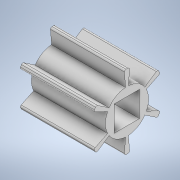
# Autodesk Inventor part: 220411 Small Rod Laddered
Saved by Autodesk Inventor 2022 (Build 260153000, 153)
## iProperties
Created: 2022-01-22
Part Number: 220411 Small Rod Laddered
Material: Generic
Document SubType Name: Modeling
Designer: josephinew
Density: 1 g/cm^3
Appearance: Default
Author: josephinew
Autodesk Inventor part; units mm, degrees
ref_plane "YZ Plane" through (0, 0, 0) normal (1, 0, 0) x (0, 1, 0)
ref_plane "XZ Plane" through (0, 0, 0) normal (0, 1, 0) x (-1, 0, 0)
ref_plane "XY Plane" through (0, 0, 0) normal (0, 0, 1) x (1, 0, 0)
sketch "Sketch1" plane through (0, 0, 0) normal (1, 0, 0) x (0, 1, 0)
  circle A0 centre (0, 0) radius 22.225
  line L0 (13.208, 13.208) -> (-12.954, 13.208)
  line L1 (-12.954, 13.208) -> (-12.954, -12.954)
  line L2 (-12.954, -12.954) -> (13.208, -12.954)
  line L3 (13.208, -12.954) -> (13.208, 13.208)
  dimension "d22" = 44.45
  dimension "d47" = 26.162
  dimension "d48" = 26.162
  constraints: 8 end point, 2 parallel, 1 centre point, 1 horizontal, 1 perpendicular
  measures "d22" diameter of A0
  measures "d47" distance of L2.end L1.end
  measures "d48" distance of L1.end L0.end
extrude "Extrusion1" add sketch "Sketch1" along normal blind 76.2
sketch "Sketch5" plane through (76.2, 0, 0) normal (1, 0, 0) x (0, 0, -1)
  line L0 (0, 0) -> (28.6448, 0) construction
  line L1 (0, 0) -> (30.2362, 0) construction
  arc A0 (0.897, 25.3842) -> (-0.897, 25.3842) centre (0, 0) ccw
  arc A1 (1.7718, 25.3381) -> (-1.7718, 25.3381) centre (0, 0) ccw
  line L2 (1.7718, 25.3381) -> (2.1549, 30.8165)
  line L3 (0, 0) -> (34.3869, 0) construction
  line L4 (0, 0) -> (33.5211, 0) construction
  line L5 (-1.7718, 25.3381) -> (-2.136, 30.8202)
  line L6 (0, 0) -> (34.3869, 0) construction
  arc A2 (1.0027, 38.0868) -> (-1.0027, 38.0868) centre (0, 0) ccw
  line L7 (1.7718, 25.3381) -> (2.5446, 36.3891)
  line L8 (-1.7718, 25.3381) -> (-2.5446, 36.3891)
  arc A3 (1.7718, 25.3381) -> (-1.7718, 25.3381) centre (0, 0) ccw
  arc A4 (-1.0027, 38.0868) -> (-2.5446, 36.3891) centre (-0.9609, 36.4999) ccw
  arc A5 (2.5446, 36.3891) -> (1.0027, 38.0868) centre (0.9609, 36.4999) ccw
  point P0 (-1.7718, 25.3381)
  point P1 (2.2148, 31.6727)
  point P2 (-2.1928, 31.6742)
  point P3 (-0.897, 25.3842)
  point P4 (0.897, 25.3842)
  point P5 (2.6577, 38.0072)
  point P6 (-2.6577, 38.0072)
  dimension "d53" = 76.2
  dimension "d54" = 1.5875
  constraints: 18 end point, 16 point on circle, 6 centre point, 5 coincident, 5 horizontal, 4 point on line, 4 tangent, 2 line through centre, 1 equal radius
  measures "d53" diameter of A2
  measures "d54" radius of A4
extrude "Extrusion4" add sketch "Sketch5" against normal blind 76.2 fills toward (-2.1083, 30.8671) open curves L8 A4 A2 A5 L7
pattern_circular "Circular Pattern1" count 6 over 360 about axis through (0, 0, 0) along (1, 0, 0) of "Extrusion4"
body "Solid1"
